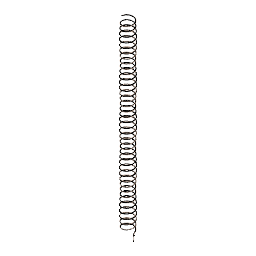
Winding Clamp (Autodesk Fusion 360 archive; units mm, degrees)
design "Copper Wire"
part number: 2026-03-20-11-23-08-707
Autodesk Fusion 360 part; units mm, degrees
(part 1 of 5)
coil "Grundkörper Spirale1" add diameter 98.84 section triangle out size 5 inside turns 39.5 pitch 39.502 right hand placed x (1, 0, 0) y (0, 1, 0) z (0, 0, 1) at (0, 0, 0) makes body 1
sketch "Skizze7" plane through (0, 0, 0) normal (0, 0, 1) x (1, 0, 0)
  line L0 (49.42, 0, 0) -> (49.42, 0, -20)
  line L1 (49.42, 0, -20) -> (49.42, 0, -60)
  line L2 (49.42, 0, 0) -> (45.4352, 19.4331, 2.5409)